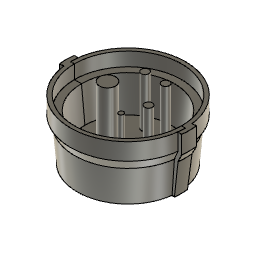
Molde tampa silicone GL80 v11 (Autodesk Fusion 360 design; units mm, degrees)
Autodesk Fusion 360 part; units mm, degrees
sketch "paredes" plane through (0, 0, 0) normal (0, 1, 0) x (1, 0, 0)
  line L0 (42, -10) -> (39.2, -10)
  line L1 (31.5, 25) -> (34, 28)
  line L2 (42, 4.4829) -> (42, -10)
  line L3 (31.5, 25) -> (34, -0.0278)
  line L4 (0, 33) -> (0, 25)
  line L5 (0, -10) -> (39.2, -10)
  line L6 (34, 28) -> (34, 30)
  line L7 (0, 0) -> (0, -10)
  line L8 (39.2, -0.0278) -> (39.2, -10)
  line L9 (0, 25) -> (31.5, 25)
  line L10 (0, 0) -> (0, 25)
  line L11 (34, 30) -> (31.5, 33)
  line L12 (34, -0.0278) -> (39.2, -0.0278)
  line L13 (0, 33) -> (37.0484, 33)
  line L14 (42, 4.4829) -> (42, 2.3652)
  line L15 (42, 2.3652) -> (38.9485, 9.063)
  line L16 (38.9485, 9.063) -> (37.0484, 33)
  line L17 (42, -10) -> (45, -10)
  line L18 (45, -10) -> (45, 3)
  line L19 (45, 3) -> (42, 9)
  line L20 (42, 9) -> (39, 33)
  line L21 (39, 33) -> (37.0484, 33)
  point P0 (38.9485, 9.063)
  dimension "d5" = 34
  dimension "d6" = 25
  dimension "d7" = 31.5
  constraint coincident L7.start L10.start
  constraint perpendicular L9 L10
  constraint perpendicular L8 L12
  constraint parallel L7 L10
  constraint perpendicular L5 L8
  constraint horizontal L13
  constraint perpendicular L2 L12
  constraint perpendicular L4 L9
  constraint perpendicular L6 L9
  constraint coincident L11.end L13
  constraint coincident P0 L15.end
  constraint coincident L2 L14.end
  constraint horizontal L5
  constraint perpendicular L2 L17
  constraint perpendicular L17 L18
  constraint parallel L13 L21
  measures "d5" distance of L3.end L7.start
  measures "d6" distance of L7.start L4.end
  measures "d7" distance of L4.end L1.start
revolve "Revolve1" add sketch "paredes" angle 360 about axis through (0, 0, -33) along (0, 0, 1) contours L1 L4 L6 L9 L11 L13 makes body 1
revolve "Revolve2" add sketch "paredes" angle 180 about axis through (0, 0, 0) along (0, 0, 1) separate body contours L0 L1 L2 L3 L6 L8 L11 L12 L13 L15 L16 makes body 2
sketch "base e furos" plane through (0, 0, -25) normal (0, 0, 1) x (-1, 0, 0)
  circle A0 centre (0, 0) radius 31.5
  circle A1 centre (7.5, -20) radius 2.825
  circle A2 centre (-7.5, -20) radius 2.825
  circle A3 centre (15, 0) radius 5.9
  circle A4 centre (-15, 0) radius 2.825
  circle A5 centre (-10, 15) radius 1.825
  dimension "d15" = 5.65
  dimension "d17" = 5.65
  dimension "d18" = 11.8
  dimension "d31" = 5.65
  dimension "d32" = 3.65
  measures "d15" diameter of A1
  measures "d17" diameter of A2
  measures "d18" diameter of A3
  measures "d31" diameter of A4
  measures "d32" diameter of A5
copy_body "CopyPasteBodies1" bodies 2 makes body 3
revolve "Revolve3" add sketch "paredes" angle 7 about axis through (0, 0, 0) along (0, 0, 1) second angle 7 contours L2 L15 L16 L17 L18 L19 L20 L21 bodies 2 3
copy_body "CopyPasteBodies3" bodies 2 makes body 4
move_body "Move3" bodies 4 to x (-1, 0, 0) y (0, -1, 0) z (0, 0, 1) at (0, 0, 0)
extrude "Extrude2" add sketch "base e furos" along normal blind 36 contours A1 | A2 | A3 | A4 | A5 bodies 1
named bodies: "base", "parede", "parede 1", "parede"
